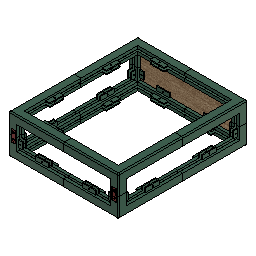
Frame_v46 (Autodesk Fusion 360 design; units mm, degrees)
Autodesk Fusion 360 part; units mm, degrees
(part 1 of 4)
sketch "Esquisse1" plane through (0, 0, 0) normal (0, 0, 1) x (1, 0, 0) in component "Wood_Bottom"
  line L0 (-125, 150) -> (125, 150)
  line L1 (125, 150) -> (125, -150)
  line L2 (125, -150) -> (-125, -150)
  line L3 (-125, -150) -> (-125, 150)
  line L4 (0, 150) -> (0, -150) construction
  line L5 (-125, 0) -> (125, 0) construction
  dimension "d4" = 250
  dimension "d5" = 300
  constraint horizontal L0
  constraint vertical L1
  constraint horizontal L2
  constraint vertical L3
  constraint midpoint L0 L4.start
  constraint midpoint L2 L4.end
  constraint midpoint L3 L5.start
  constraint midpoint L1 L5.end
  constraint midpoint L4 origin
  measures "d4" distance of L0.start L0.end
  measures "d5" distance of L0.start L2.end
extrude "Extrusion1" add sketch "Esquisse1" along normal blind 5 makes body 1 in component "Wood_Bottom"
sketch "Esquisse1 (2)" plane through (0, 0, 0) normal (1, 0, 0) x (0, 1, 0) in component "Right_Bottom_Holder"
  line L0 (-165, 59.7937) -> (165, 59.7937)
  line L1 (165, 59.7937) -> (165, 39.4937)
  line L2 (165, 39.4937) -> (-165, 39.4937)
  line L3 (-165, 39.4937) -> (-165, 59.7937)
  line L4 (0, 59.7937) -> (0, 39.4937) construction
  line L5 (-165, 49.6437) -> (165, 49.6437) construction
  point P0 (0, 49.6437)
  dimension "d11" = 330
  dimension "d12" = 20.3
  constraint horizontal L0
  constraint vertical L1
  constraint horizontal L2
  constraint vertical L3
  constraint midpoint L0 L4.start
  constraint midpoint L2 L4.end
  constraint midpoint L3 L5.start
  constraint midpoint L1 L5.end
  constraint midpoint L5 P0
  constraint vertical origin P0
  measures "d11" distance of L0.start L0.end
  measures "d12" distance of L0.start L2.end
extrude "Extrusion1'" add sketch "Esquisse1 (2)" along normal blind 20 separate body makes body 2 in component "Right_Bottom_Holder"
sketch "Esquisse2" plane through (0, 0, 0) normal (-1, 0, 0) x (0, -1, 0) in component "Right_Bottom_Holder"
  line L0 (-165, 39.4937) -> (165, 39.4937)
  line L1 (165, 39.4937) -> (165, 59.7937)
  line L2 (165, 59.7937) -> (-165, 59.7937)
  line L3 (-165, 59.7937) -> (-165, 39.4937)
  line L4 (-150.3, 52.4437) -> (150.3, 52.4437)
  line L5 (150.3, 52.4437) -> (150.3, 46.8437)
  line L6 (150.3, 46.8437) -> (-150.3, 46.8437)
  line L7 (-150.3, 46.8437) -> (-150.3, 52.4437)
  line L8 (-165, 49.6437) -> (165, 49.6437) construction
  line L9 (0, 59.7937) -> (0, 39.4937) construction
  line L10 (-165, 59.7937) -> (-145, 59.7937)
  line L11 (-145, 59.7937) -> (-145, 39.4937)
  line L12 (-145, 39.4937) -> (-165, 39.4937)
  line L13 (-165, 39.4937) -> (-165, 59.7937)
  line L14 (165, 59.7937) -> (145, 59.7937)
  line L15 (145, 59.7937) -> (145, 39.4937)
  line L16 (145, 39.4937) -> (165, 39.4937)
  line L17 (165, 39.4937) -> (165, 59.7937)
  line L18 (90, 52.4437) -> (55, 52.4437)
  line L19 (55, 52.4437) -> (55, 54.9437)
  line L20 (55, 54.9437) -> (90, 54.9437)
  line L21 (90, 54.9437) -> (90, 52.4437)
  line L22 (90, 54.9437) -> (145, 54.9437) construction
  line L23 (55, 54.9437) -> (0, 54.9437) construction
  line L24 (90, 46.8437) -> (55, 46.8437)
  line L25 (90, 44.3437) -> (90, 46.8437)
  line L26 (55, 46.8437) -> (55, 44.3437)
  line L27 (55, 44.3437) -> (90, 44.3437)
  line L28 (-55, 46.8437) -> (-55, 44.3437)
  line L29 (-90, 54.9437) -> (-90, 52.4437)
  line L30 (-55, 52.4437) -> (-55, 54.9437)
  line L31 (-55, 54.9437) -> (-90, 54.9437)
  line L32 (-90, 44.3437) -> (-90, 46.8437)
  line L33 (-90, 46.8437) -> (-55, 46.8437)
  line L34 (-55, 44.3437) -> (-90, 44.3437)
  line L35 (-90, 52.4437) -> (-55, 52.4437)
  point P0 (150.3, 49.6437)
  point P1 (0, 52.4437)
  point P2 (0, 53.6937)
  dimension "d16" = 5.6
  dimension "d17" = 300.6
  dimension "d109" = 20
  dimension "d110" = 20.3
  dimension "d111" = 20
  dimension "d112" = 20.3
  dimension "d230" = 2.5
  dimension "d231" = 35
  constraint horizontal L4
  constraint vertical L5
  constraint horizontal L6
  constraint vertical L7
  constraint midpoint L3 L8.start
  constraint midpoint L1 L8.end
  constraint midpoint L5 P0
  constraint coincident L8 P0
  constraint midpoint L4 P1
  constraint midpoint L2 L9.start
  constraint midpoint L0 L9.end
  constraint coincident P1 L9
  constraint coincident L9 P2
  constraint horizontal L10
  constraint vertical L11
  constraint horizontal L12
  constraint vertical L13
  constraint coincident L2.end L3.start
  constraint horizontal L14
  constraint vertical L15
  constraint horizontal L16
  constraint vertical L17
  constraint coincident L1.end L2.start
  constraint horizontal L18
  constraint vertical L19
  constraint horizontal L20
  constraint vertical L21
  constraint coincident L4 L18.start
  constraint coincident L15 L22.end
  constraint perpendicular L15 L22
  constraint coincident L9 L23.end
  constraint perpendicular L9 L23
  constraint equal L22 L23
  constraint symmetric L8 L18.start L24.start
  constraint symmetric L8 L18.end L24.end
  constraint symmetric L8 L19.end L26.end
  constraint symmetric L8 L20.end L25.start
  constraint symmetric L9 L18.start L29.end
  constraint symmetric L9 L18.end L30.start
  constraint symmetric L9 L19.end L30.end
  constraint symmetric L9 L20.end L29.start
  constraint symmetric L9 L24.start L32.end
  constraint symmetric L9 L24.end L28.start
  constraint symmetric L9 L25.start L32.start
  constraint symmetric L9 L26.end L28.end
  measures "d16" distance of L4 L6
  measures "d17" distance of L4.start L4.end
  measures "d109" distance of L2.end L10.end
  measures "d110" distance of L10.end L11.end
  measures "d111" distance of L1.end L14.end
  measures "d112" distance of L14.end L15.end
  measures "d230" distance of L18.start L20.end
  measures "d231" distance of L19.end L20.end
extrude "Extrusion2" cut sketch "Esquisse2" against normal blind 5 contours L4 L6 L11 L15 L18 L24 L33 L35 | L4 L6 L7 L11 | L4 L5 L6 L15 bodies 2 in component "Right_Bottom_Holder"
extrude "Extrusion3" add sketch "Esquisse2" along normal blind 10 contours L6 L28 L32 L33 L34 | L6 L24 L25 L26 L27 | L4 L29 L30 L31 L35 | L4 L18 L19 L20 L21 bodies 2 in component "Right_Bottom_Holder"
extrude "Extrusion19" add sketch "Esquisse2" along normal blind 120.3 contours L0 L2 L3 L4 L6 L7 L10 L11 L12 L13 | L0 L1 L2 L4 L5 L6 L14 L15 L16 L17 bodies 2 in component "Right_Bottom_Holder"
sketch "Esquisse14" plane through (-120.3, 0, 0) normal (-1, 0, 0) x (0, -1, 0) in component "Right_Bottom_Holder"
  line L0 (-145, 46.8437) -> (-150.3, 46.8437)
  line L1 (-150.3, 46.8437) -> (-150.3, 52.4437)
  line L2 (-150.3, 52.4437) -> (-145, 52.4437)
  line L3 (-145, 52.4437) -> (-145, 59.7937)
  line L4 (-145, 59.7937) -> (-165, 59.7937)
  line L5 (-165, 59.7937) -> (-165, 39.4937)
  line L6 (-165, 39.4937) -> (-145, 39.4937)
  line L7 (-145, 39.4937) -> (-145, 46.8437)
  line L8 (-155, 59.7937) -> (-155, 39.4937) construction
  line L9 (-165, 49.6437) -> (-155, 49.6437) construction
  line L10 (-165, 49.6437) -> (-155, 39.4937) construction
  line L11 (-165, 39.4937) -> (-155, 49.6437) construction
  circle A0 centre (-160, 44.5687) radius 2.65
  line L12 (-157.8, 59.7937) -> (-152.2, 59.7937)
  line L13 (-152.2, 59.7937) -> (-152.2, 54.4937)
  line L14 (-152.2, 54.4937) -> (-157.8, 54.4937)
  line L15 (-157.8, 54.4937) -> (-157.8, 59.7937)
  point P0 (-155, 54.4937)
  dimension "d117" = 5.3
  dimension "d118" = 5.6
  dimension "d119" = 5.3
  constraint midpoint L4 L8.start
  constraint midpoint L6 L8.end
  constraint midpoint L5 L9.start
  constraint midpoint L8 L9.end
  constraint coincident L5.end L6.start
  constraint midpoint L10 A0.centre
  constraint horizontal L12
  constraint vertical L13
  constraint horizontal L14
  constraint vertical L15
  constraint coincident L4 L12.start
  constraint midpoint L14 P0
  constraint coincident L8 P0
  measures "d117" diameter of A0
  measures "d118" distance of L13.end L14.end
  measures "d119" distance of L12.end L13.end
extrude "Extrusion20" cut sketch "Esquisse14" against normal blind 10.3 contours A0 bodies 2 in component "Right_Bottom_Holder"
extrude "Extrusion21" cut sketch "Esquisse14" against normal up to surface (125.6 mm away) contours L4 L12 L13 L14 L15 bodies 2 in component "Right_Bottom_Holder"
sketch "Esquisse15" plane through (0, 145, 0) normal (0, -1, 0) x (1, 0, 0) in component "Right_Bottom_Holder"
  line L0 (0, 52.4437) -> (0, 59.7937)
  line L1 (0, 59.7937) -> (-120.3, 59.7937)
  line L2 (-120.3, 59.7937) -> (-120.3, 52.4437)
  line L3 (-120.3, 52.4437) -> (0, 52.4437)
  line L4 (0, 46.8437) -> (-120.3, 46.8437)
  line L5 (-120.3, 46.8437) -> (-120.3, 39.4937)
  line L6 (-120.3, 39.4937) -> (0, 39.4937)
  line L7 (-60.15, 59.7937) -> (-60.15, 52.4437) construction
  line L8 (-60.15, 52.4437) -> (-60.15, 46.8437) construction
  line L9 (-60.15, 49.6437) -> (-55, 49.6437) construction
  line L10 (-77.65, 52.4437) -> (-42.65, 52.4437)
  line L11 (-42.65, 52.4437) -> (-42.65, 54.9437)
  line L12 (-42.65, 54.9437) -> (-77.65, 54.9437)
  line L13 (-77.65, 54.9437) -> (-77.65, 52.4437)
  line L14 (-42.65, 44.3437) -> (-77.65, 44.3437)
  line L15 (-77.65, 44.3437) -> (-77.65, 46.8437)
  line L16 (-77.65, 46.8437) -> (-42.65, 46.8437)
  line L17 (-42.65, 46.8437) -> (-42.65, 44.3437)
  line L18 (0, 39.4937) -> (0, 46.8437)
  point P0 (-60.15, 54.9437)
  dimension "d124" = 2.5
  dimension "d125" = 35
  constraint midpoint L1 L7.start
  constraint midpoint L3 L7.end
  constraint midpoint L4 L8.end
  constraint midpoint L8 L9.start
  constraint perpendicular L8 L9
  constraint horizontal L10
  constraint vertical L11
  constraint horizontal L12
  constraint vertical L13
  constraint coincident L3 L10.start
  constraint midpoint L12 P0
  constraint coincident L7 P0
  constraint symmetric L9 L10.start L15.end
  constraint symmetric L9 L10.end L16.end
  constraint symmetric L9 L11.end L14.start
  constraint symmetric L9 L12.end L14.end
  measures "d124" distance of L10.end L11.end
  measures "d125" distance of L11.end L12.end
extrude "Extrusion22" add sketch "Esquisse15" along normal blind 10 contours L3 L10 L11 L12 L13 | L4 L14 L15 L16 L17 bodies 2 in component "Right_Bottom_Holder"
sketch "Esquisse17" plane through (-120.3, 0, 0) normal (-1, 0, 0) x (0, -1, 0) in component "Right_Bottom_Holder"
  line L0 (165, 39.4937) -> (165, 59.7937)
  line L1 (165, 59.7937) -> (145, 59.7937)
  line L2 (145, 59.7937) -> (145, 52.4437)
  line L3 (145, 52.4437) -> (150.3, 52.4437)
  line L4 (150.3, 52.4437) -> (150.3, 46.8437)
  line L5 (150.3, 46.8437) -> (145, 46.8437)
  line L6 (145, 46.8437) -> (145, 39.4937)
  line L7 (145, 39.4937) -> (165, 39.4937)
  line L8 (155, 59.7937) -> (155, 39.4937) construction
  line L9 (165, 49.6437) -> (145, 49.6437) construction
  line L10 (155, 49.6437) -> (165, 39.4937) construction
  line L11 (155, 39.4937) -> (165, 49.6437) construction
  circle A0 centre (160, 44.5687) radius 2.65
  line L12 (152.2, 59.7937) -> (157.8, 59.7937)
  line L13 (157.8, 59.7937) -> (157.8, 54.4937)
  line L14 (157.8, 54.4937) -> (152.2, 54.4937)
  line L15 (152.2, 54.4937) -> (152.2, 59.7937)
  point P0 (155, 54.4937)
  dimension "d134" = 5.3
  dimension "d135" = 5.3
  dimension "d136" = 5.6
  constraint midpoint L1 L8.start
  constraint midpoint L7 L8.end
  constraint midpoint L0 L9.start
  constraint perpendicular L2 L9
  constraint midpoint L8 L10.start
  constraint coincident L0.start L7.end
  constraint midpoint L10 A0.centre
  constraint horizontal L12
  constraint vertical L13
  constraint horizontal L14
  constraint vertical L15
  constraint coincident L1 L12.start
  constraint midpoint L14 P0
  constraint coincident L8 P0
  measures "d134" diameter of A0
  measures "d135" distance of L12.end L13.end
  measures "d136" distance of L13.end L14.end
extrude "Extrusion25" cut sketch "Esquisse17" against normal blind 10.3 contours A0 bodies 2 in component "Right_Bottom_Holder"
extrude "Extrusion26" cut sketch "Esquisse17" against normal up to surface (125.6 mm away) contours L1 L12 L13 L14 L15 bodies 2 in component "Right_Bottom_Holder"
sketch "Esquisse18" plane through (0, -145, 0) normal (0, 1, 0) x (-1, 0, 0) in component "Right_Bottom_Holder"
  line L0 (0, 59.7937) -> (0, 52.4437)
  line L1 (0, 52.4437) -> (120.3, 52.4437)
  line L2 (120.3, 52.4437) -> (120.3, 59.7937)
  line L3 (120.3, 59.7937) -> (0, 59.7937)
  line L4 (0, 39.4937) -> (120.3, 39.4937) construction
  line L5 (120.3, 39.4937) -> (120.3, 46.8437) construction
  line L6 (120.3, 46.8437) -> (0, 46.8437) construction
  line L7 (60.15, 59.7937) -> (60.15, 52.4437) construction
  line L8 (60.15, 52.4437) -> (60.15, 46.8437) construction
  line L9 (60.15, 49.6437) -> (66.8882, 49.6437) construction
  line L10 (42.65, 52.4437) -> (77.65, 52.4437)
  line L11 (77.65, 52.4437) -> (77.65, 54.9437)
  line L12 (77.65, 54.9437) -> (42.65, 54.9437)
  line L13 (42.65, 54.9437) -> (42.65, 52.4437)
  line L14 (77.65, 44.3437) -> (42.65, 44.3437)
  line L15 (77.65, 46.8437) -> (77.65, 44.3437)
  line L16 (42.65, 44.3437) -> (42.65, 46.8437)
  line L17 (42.65, 46.8437) -> (77.65, 46.8437)
  line L18 (0, 46.8437) -> (0, 39.4937)
  point P0 (60.15, 54.9437)
  dimension "d141" = 2.5
  dimension "d142" = 35
  constraint midpoint L3 L7.start
  constraint midpoint L1 L7.end
  constraint midpoint L6 L8.end
  constraint midpoint L8 L9.start
  constraint perpendicular L8 L9
  constraint horizontal L10
  constraint vertical L11
  constraint horizontal L12
  constraint vertical L13
  constraint coincident L1 L10.start
  constraint midpoint L12 P0
  constraint coincident L7 P0
  constraint symmetric L9 L10.start L16.end
  constraint symmetric L9 L10.end L15.start
  constraint symmetric L9 L11.end L14.start
  constraint symmetric L9 L12.end L14.end
  measures "d141" distance of L10.end L11.end
  measures "d142" distance of L11.end L12.end
extrude "Extrusion27" add sketch "Esquisse18" along normal blind 10 contours L1 L10 L11 L12 L13 | L14 L15 L16 L17 bodies 2 in component "Right_Bottom_Holder"
sketch "Esquisse16" plane through (0, 0, 59.7937) normal (0, 0, 1) x (-1, 0, 0) in component "Right_Bottom_Holder"
  line L0 (-5.3, -152.2) -> (120.3, -152.2)
  line L1 (120.3, -152.2) -> (120.3, -145)
  line L2 (120.3, -145) -> (0, -145)
  line L3 (0, -145) -> (0, 145)
  line L4 (0, 145) -> (120.3, 145)
  line L5 (120.3, 157.8) -> (120.3, 165)
  line L6 (120.3, 165) -> (-20, 165)
  line L7 (-20, 165) -> (-20, -165)
  line L8 (-20, -165) -> (120.3, -165)
  line L9 (120.3, -165) -> (120.3, -157.8)
  line L10 (120.3, -157.8) -> (-5.3, -157.8)
  line L11 (-5.3, -157.8) -> (-5.3, -152.2)
  line L12 (0.0045, -165) -> (120.3, -165) construction
  line L13 (60.1522, -165) -> (60.15, -145) construction
  line L14 (60.1511, -155) -> (47.2609, -155.0014) construction
  line L15 (77.6517, -157.8) -> (42.6517, -157.8)
  line L16 (42.6517, -157.8) -> (42.6517, -160.3)
  line L17 (42.6517, -160.3) -> (77.6517, -160.3)
  line L18 (77.6517, -160.3) -> (77.6517, -157.8)
  line L19 (77.6505, -149.6961) -> (77.6511, -152.1961)
  line L20 (42.6505, -149.7039) -> (77.6505, -149.6961)
  line L21 (77.6511, -152.1961) -> (42.6511, -152.2039)
  line L22 (42.6511, -152.2039) -> (42.6505, -149.7039)
  line L23 (0, -145) -> (-20, -145)
  line L24 (-20, -145) -> (-20, -165)
  line L25 (-20, -165) -> (0, -165)
  line L26 (0, -165) -> (0, -145)
  line L27 (-20, 0) -> (0, 0) construction
  line L28 (-12.8, -150.3) -> (-7.2, -150.3)
  line L29 (-7.2, -150.3) -> (-7.2, 150.3)
  line L30 (-7.2, 150.3) -> (-12.8, 150.3)
  line L31 (-12.8, 150.3) -> (-12.8, -150.3)
  line L32 (-10, -165) -> (-10, -145) construction
  line L33 (0, 145) -> (-20, 145)
  line L34 (-20, 145) -> (-20, 165)
  line L35 (-20, 165) -> (0, 165)
  line L36 (0, 165) -> (0, 145)
  line L37 (-12.8, 70) -> (-12.8, -70)
  line L38 (-10, 0) -> (-10, 10) construction
  line L39 (-7.2, 70) -> (-7.2, -70)
  line L40 (0, 165) -> (120.3, 165) construction
  line L41 (60.15, 165) -> (60.15, 145) construction
  line L42 (-5.3, 157.8) -> (120.3, 157.8)
  line L43 (120.3, 152.2) -> (-5.3, 152.2)
  line L44 (-5.3, 152.2) -> (-5.3, 157.8)
  line L45 (-5.3, 157.8) -> (-5.3, 152.2)
  line L46 (-5.3, 152.2) -> (120.3, 152.2)
  line L47 (120.3, 152.2) -> (120.3, 157.8)
  line L48 (120.3, 157.8) -> (-5.3, 157.8)
  line L49 (42.65, 157.8) -> (77.65, 157.8)
  line L50 (77.65, 157.8) -> (77.65, 160.3)
  line L51 (77.65, 160.3) -> (42.65, 160.3)
  line L52 (42.65, 160.3) -> (42.65, 157.8)
  line L53 (60.15, 155) -> (66, 155) construction
  line L54 (42.65, 152.2) -> (77.65, 152.2)
  line L55 (42.65, 149.7) -> (42.65, 152.2)
  line L56 (77.65, 149.7) -> (42.65, 149.7)
  line L57 (77.65, 152.2) -> (77.65, 149.7)
  line L58 (-12.8, -90) -> (-15.3, -90)
  line L59 (-15.3, -90) -> (-15.3, -55)
  line L60 (-15.3, -55) -> (-12.8, -55)
  line L61 (-12.8, -55) -> (-12.8, -90)
  line L62 (-15.3, -90) -> (-15.3, -145) construction
  line L63 (-15.3, -55) -> (-15.3, 0) construction
  line L64 (-4.7, -90) -> (-4.7, -55)
  line L65 (-4.7, -55) -> (-7.2, -55)
  line L66 (-7.2, -90) -> (-4.7, -90)
  line L67 (-7.2, -55) -> (-7.2, -90)
  line L68 (-7.2, 55) -> (-7.2, 90)
  line L69 (-12.8, 55) -> (-12.8, 90)
  line L70 (-15.3, 55) -> (-12.8, 55)
  line L71 (-15.3, 90) -> (-15.3, 55)
  line L72 (-12.8, 90) -> (-15.3, 90)
  line L73 (-7.2, 90) -> (-4.7, 90)
  line L74 (-4.7, 90) -> (-4.7, 55)
  line L75 (-4.7, 55) -> (-7.2, 55)
  point P0 (60.1517, -160.3)
  point P1 (-10, -150.3)
  point P2 (-12.8, 0)
  point P3 (-15.3, 0)
  point P4 (60.15, 160.3)
  dimension "d128" = 2.5
  dimension "d129" = 35
  dimension "d145" = 5.6
  dimension "d146" = 300.6
  dimension "d149" = 2.5
  dimension "d150" = 35
  dimension "d232" = 2.5
  dimension "d233" = 35
  constraint coincident L8 L12.start
  constraint coincident L8.end L9.start
  constraint midpoint L12 L13.start
  constraint midpoint L2 L13.end
  constraint midpoint L13 L14.start
  constraint perpendicular L13 L14
  constraint horizontal L15
  constraint vertical L16
  constraint horizontal L17
  constraint vertical L18
  constraint coincident L10 L15.start
  constraint midpoint L17 P0
  constraint coincident L13 P0
  constraint symmetric L14 L15.start L19.end
  constraint symmetric L14 L15.end L21.end
  constraint symmetric L14 L16.end L20.start
  constraint symmetric L14 L17.end L19.start
  constraint horizontal L23
  constraint vertical L24
  constraint horizontal L25
  constraint vertical L26
  constraint coincident L7.end L8.start
  constraint coincident L2.end L3.start
  constraint midpoint L7 L27.start
  constraint coincident L27.end origin
  constraint horizontal L28
  constraint vertical L29
  constraint horizontal L30
  constraint vertical L31
  constraint midpoint L28 P1
  constraint midpoint L25 L32.start
  constraint midpoint L23 L32.end
  constraint coincident P1 L32
  constraint midpoint L31 P2
  constraint coincident L27 P2
  constraint horizontal L33
  constraint vertical L34
  constraint horizontal L35
  constraint vertical L36
  constraint coincident L6.end L7.start
  constraint coincident L3.end L4.start
  constraint vertical L37
  constraint coincident L31 L37.end
  constraint coincident L27 P3
  constraint midpoint L27 L38.start
  constraint perpendicular L27 L38
  constraint symmetric L37.end L38 L39.end
  constraint symmetric L37.start L38 L39.start
  constraint coincident L5.end L6.start
  constraint midpoint L40 L41.start
  constraint midpoint L4 L41.end
  constraint horizontal L49
  constraint vertical L50
  constraint horizontal L51
  constraint vertical L52
  constraint coincident L42 L49.start
  constraint midpoint L51 P4
  constraint coincident L41 P4
  constraint midpoint L41 L53.start
  constraint perpendicular L41 L53
  constraint symmetric L49.start L53 L54.start
  constraint symmetric L49.end L53 L54.end
  constraint symmetric L50.end L53 L56.start
  constraint symmetric L51.end L53 L55.start
  constraint horizontal L58
  constraint vertical L59
  constraint horizontal L60
  constraint vertical L61
  constraint coincident L31 L58.start
  constraint coincident L23 L62.end
  constraint perpendicular L23 L62
  constraint coincident P3 L63.end
  constraint perpendicular L27 L63
  constraint equal L62 L63
  constraint symmetric L38 L58.start L66.start
  constraint symmetric L38 L58.end L64.start
  constraint symmetric L38 L59.end L64.end
  constraint symmetric L38 L60.end L65.end
  constraint symmetric L27 L58.start L69.end
  constraint symmetric L27 L58.end L71.start
  constraint symmetric L27 L59.end L70.start
  constraint symmetric L27 L60.end L69.start
  constraint symmetric L27 L64.start L73.end
  constraint symmetric L27 L64.end L74.end
  constraint symmetric L27 L65.end L68.start
  constraint symmetric L27 L66.start L68.end
  measures "d128" distance of L15.end L16.end
  measures "d129" distance of L16.end L17.end
  measures "d145" distance of L28.start L28.end
  measures "d146" distance of L28.start L30.end
  measures "d149" distance of L49.start L51.end
  measures "d150" distance of L50.end L51.end
  measures "d232" distance of L58.start L58.end
  measures "d233" distance of L58.end L59.end
extrude "Extrusion23" add sketch "Esquisse16" along normal blind 10 contours L0 L19 L20 L21 L22 | L0 L21 L22 | L10 L15 L16 L17 L18 | L29 L39 L64 L65 L66 L67 | L29 L39 L68 L73 L74 L75 | L43 L46 L54 L55 L56 L57 | L31 L37 L58 L59 L60 L61 | L31 L37 L69 L70 L71 L72 | L42 L48 L49 L50 L51 L52 bodies 2 in component "Right_Bottom_Holder"
extrude "Extrusion28" cut sketch "Esquisse16" against normal blind 5.3 contours L23 L28 L29 L31 | L23 L29 L31 L33 L37 L39 L61 L67 L68 L69 | L29 L30 L31 L33 bodies 2 in component "Right_Bottom_Holder"
extrude "Extrusion29" add sketch "Esquisse16" along normal blind 30 contours L0 L7 L8 L10 L11 L23 L24 L25 L26 L28 L29 L31 | L6 L7 L29 L30 L31 L33 L34 L35 L36 L42 L43 L44 L45 L46 L48 bodies 2 in component "Right_Bottom_Holder"
sketch "Esquisse20" plane through (0, 0, 89.7937) normal (0, 0, 1) x (-1, 0, 0) in component "Right_Bottom_Holder"
  line L0 (0, 165) -> (-20, 165)
  line L1 (-20, 165) -> (-20, 145)
  line L2 (-20, 145) -> (-12.8, 145)
  line L3 (-12.8, 145) -> (-12.8, 150.3)
  line L4 (-12.8, 150.3) -> (-7.2, 150.3)
  line L5 (-7.2, 150.3) -> (-7.2, 145)
  line L6 (-7.2, 145) -> (0, 145)
  line L7 (0, 145) -> (0, 152.2)
  line L8 (0, 152.2) -> (-5.3, 152.2)
  line L9 (-5.3, 152.2) -> (-5.3, 157.8)
  line L10 (-5.3, 157.8) -> (0, 157.8)
  line L11 (0, 157.8) -> (0, 165)
  line L12 (-20, 155) -> (0, 155) construction
  line L13 (-10, 165) -> (-10, 145) construction
  circle A0 centre (-15, 155) radius 2.5
  line L14 (-20, 145) -> (0, 145) construction
  line L15 (-20, 165) -> (-10, 165) construction
  line L16 (-15, 165) -> (-15, 145) construction
  line L17 (-12.8, -150.3) -> (-12.8, -145)
  line L18 (-12.8, -145) -> (-20, -145)
  line L19 (-20, -145) -> (-20, -165)
  line L20 (-20, -165) -> (0, -165)
  line L21 (0, -165) -> (0, -157.8)
  line L22 (0, -157.8) -> (-5.3, -157.8)
  line L23 (-5.3, -157.8) -> (-5.3, -152.2)
  line L24 (-5.3, -152.2) -> (0, -152.2)
  line L25 (0, -152.2) -> (0, -145)
  line L26 (0, -145) -> (-7.2, -145)
  line L27 (-7.2, -145) -> (-7.2, -150.3)
  line L28 (-7.2, -150.3) -> (-12.8, -150.3)
  line L29 (-10, -165) -> (-10, -145) construction
  line L30 (-20, -155) -> (0, -155) construction
  line L31 (-10, -165) -> (-20, -165) construction
  line L32 (-15, -165) -> (-15, -145) construction
  circle A1 centre (-15, -155) radius 2.5
  dimension "d158" = 5
  dimension "d352" = 10
  dimension "d354" = 5
  constraint midpoint L1 L12.start
  constraint perpendicular L7 L12
  constraint midpoint L0 L13.start
  constraint perpendicular L2 L13
  constraint coincident L0.end L1.start
  constraint coincident L1.end L2.start
  constraint coincident L6.end L7.start
  constraint midpoint L15 L16.start
  constraint coincident L14 L16.end
  constraint coincident A0.centre L16
  constraint midpoint L20 L29.start
  constraint perpendicular L26 L29
  constraint midpoint L19 L30.start
  constraint perpendicular L23 L30
  constraint coincident L19.end L20.start
  constraint midpoint L31 L32.start
  constraint coincident L18 L32.end
  constraint perpendicular L18 L32
  constraint midpoint L32 A1.centre
  measures "d158" diameter of A0
  measures "d352" distance of A0.centre L15
  measures "d354" diameter of A1
extrude "Extrusion31" add sketch "Esquisse20" along normal blind 10 contours A0 | A1 bodies 2 in component "Right_Bottom_Holder"
split "Scinder1" by plane through (-120.3, 0, 47.1437) normal (0, 1, 0) bodies 2 makes body 3 at (13.3333, 103.3333, 39.4937) in component "Right_Bottom_Holder"
move_body "Déplacer1" bodies 2 to x (1, 0, 0) y (0, 1, 0) z (0, 0, 1) at (0, -80, 0) in component "Right_Bottom_Holder"
sketch "Esquisse21" plane through (0, -80, 0) normal (0, 1, 0) x (-1, 0, 0) in component "Right_Bottom_Holder"
  line L0 (-10, 39.7937) -> (-10, 54.4937) construction
  line L1 (-20, 49.7937) -> (-5, 49.7937) construction
  line L2 (-20, 49.7937) -> (-10, 39.7937) construction
  line L3 (-10, 49.7937) -> (-20, 39.7937) construction
  circle A0 centre (-15, 44.7937) radius 2.65
  line L4 (0, 39.4937) -> (0, 46.8437)
  line L5 (0, 46.8437) -> (-5, 46.8437)
  line L6 (-5, 46.8437) -> (-5, 52.4437)
  line L7 (-5, 52.4437) -> (0, 52.4437)
  line L8 (0, 52.4437) -> (0, 59.7937)
  line L9 (0, 59.7937) -> (-7.2, 59.7937)
  line L10 (-7.2, 59.7937) -> (-7.2, 54.4937)
  line L11 (-7.2, 54.4937) -> (-12.8, 54.4937)
  line L12 (-12.8, 54.4937) -> (-12.8, 59.7937)
  line L13 (-12.8, 59.7937) -> (-20, 59.7937)
  line L14 (-20, 59.7937) -> (-20, 39.4937)
  line L15 (-20, 39.4937) -> (0, 39.4937)
  dimension "d161" = 5.3
  constraint coincident L0 L3.start
  constraint coincident L1 L3.start
  constraint midpoint L3 A0.centre
  measures "d161" diameter of A0
extrude "Extrusion32" cut sketch "Esquisse21" against normal blind 10.3 contours A0 bodies 2 in component "Right_Bottom_Holder"
sketch "Esquisse22" plane through (0, 0, 0) normal (0, -1, 0) x (1, 0, 0) in component "Right_Bottom_Holder"
  line L0 (10, 39.7937) -> (10, 54.4937) construction
  line L1 (20, 49.7937) -> (5, 49.7937) construction
  line L2 (20, 39.7937) -> (10, 49.7937) construction
  line L3 (10, 39.7937) -> (20, 49.7937) construction
  circle A0 centre (15, 44.7937) radius 2.5
  line L4 (0, 46.8437) -> (0, 39.4937)
  line L5 (0, 39.4937) -> (20, 39.4937)
  line L6 (20, 39.4937) -> (20, 59.7937)
  line L7 (20, 59.7937) -> (12.8, 59.7937)
  line L8 (12.8, 59.7937) -> (12.8, 54.4937)
  line L9 (12.8, 54.4937) -> (7.2, 54.4937)
  line L10 (7.2, 54.4937) -> (7.2, 59.7937)
  line L11 (7.2, 59.7937) -> (0, 59.7937)
  line L12 (0, 59.7937) -> (0, 52.4437)
  line L13 (0, 52.4437) -> (5, 52.4437)
  line L14 (5, 52.4437) -> (5, 46.8437)
  line L15 (5, 46.8437) -> (0, 46.8437)
  dimension "d164" = 5
  constraint coincident L1 L2.end
  constraint coincident L0 L2.end
  constraint midpoint L3 A0.centre
  measures "d164" diameter of A0
extrude "Extrusion33" add sketch "Esquisse22" along normal blind 10 contours A0 bodies 3 in component "Right_Bottom_Holder"
move_body "Déplacer2" bodies 2 to x (1, 0, 0) y (0, 1, 0) z (0, 0, 1) at (0, 80, 0) in component "Right_Bottom_Holder"
sketch "Esquisse23" plane through (0, 145, 0) normal (0, -1, 0) x (1, 0, 0) in component "Right_Bottom_Holder"
  line L0 (0, 59.7937) -> (7.2, 59.7937)
  line L1 (7.2, 59.7937) -> (7.2, 89.7937)
  line L2 (7.2, 89.7937) -> (0, 89.7937)
  line L3 (0, 89.7937) -> (0, 59.7937)
  line L4 (12.8, 59.7937) -> (20, 59.7937)
  line L5 (20, 59.7937) -> (20, 89.7937)
  line L6 (20, 89.7937) -> (12.8, 89.7937)
  line L7 (12.8, 89.7937) -> (12.8, 59.7937)
  line L8 (0, 74.7937) -> (7.2, 74.7937) construction
  line L9 (7.2, 74.7937) -> (12.8, 74.7937) construction
  line L10 (10, 74.7937) -> (10, 86.5) construction
  line L11 (7.2, 66.0437) -> (4.7, 66.0437)
  line L12 (4.7, 66.0437) -> (4.7, 83.5437)
  line L13 (4.7, 83.5437) -> (7.2, 83.5437)
  line L14 (7.2, 83.5437) -> (7.2, 66.0437)
  line L15 (15.3, 66.0437) -> (15.3, 83.5437)
  line L16 (15.3, 83.5437) -> (12.8, 83.5437)
  line L17 (12.8, 83.5437) -> (12.8, 66.0437)
  line L18 (12.8, 66.0437) -> (15.3, 66.0437)
  point P0 (4.7, 74.7937)
  dimension "d171" = 2.5
  dimension "d172" = 17.5
  constraint midpoint L3 L8.start
  constraint midpoint L1 L8.end
  constraint midpoint L7 L9.end
  constraint midpoint L9 L10.start
  constraint perpendicular L9 L10
  constraint horizontal L11
  constraint vertical L12
  constraint horizontal L13
  constraint vertical L14
  constraint coincident L1 L11.start
  constraint midpoint L12 P0
  constraint coincident L8 P0
  constraint symmetric L10 L11.start L17.end
  constraint symmetric L10 L11.end L15.start
  constraint symmetric L10 L12.end L15.end
  constraint symmetric L10 L13.end L16.end
  measures "d171" distance of L12.end L13.end
  measures "d172" distance of L11.end L12.end
extrude "Extrusion35" add sketch "Esquisse23" along normal blind 10 contours L1 L11 L12 L13 L14 | L7 L15 L16 L17 L18 bodies 3 in component "Right_Bottom_Holder"
sketch "Esquisse24" plane through (0, -145, 0) normal (0, 1, 0) x (-1, 0, 0) in component "Right_Bottom_Holder"
  line L0 (-20, 59.7937) -> (-12.8, 59.7937)
  line L1 (-12.8, 59.7937) -> (-12.8, 89.7937)
  line L2 (-12.8, 89.7937) -> (-20, 89.7937)
  line L3 (-20, 89.7937) -> (-20, 59.7937)
  line L4 (-20, 74.7937) -> (-12.8, 74.7937) construction
  line L5 (-7.2, 59.7937) -> (0, 59.7937) construction
  line L6 (0, 59.7937) -> (0, 89.7937) construction
  line L7 (0, 89.7937) -> (-7.2, 89.7937) construction
  line L8 (-7.2, 89.7937) -> (-7.2, 59.7937) construction
  line L9 (-12.8, 74.7937) -> (-7.2, 74.7937) construction
  line L10 (-10, 74.7937) -> (-10, 87.5) construction
  line L11 (-12.8, 66.0437) -> (-15.3, 66.0437)
  line L12 (-15.3, 66.0437) -> (-15.3, 83.5437)
  line L13 (-15.3, 83.5437) -> (-12.8, 83.5437)
  line L14 (-12.8, 83.5437) -> (-12.8, 66.0437)
  line L15 (-4.7, 66.0437) -> (-4.7, 83.5437)
  line L16 (-4.7, 83.5437) -> (-7.2, 83.5437)
  line L17 (-7.2, 83.5437) -> (-7.2, 66.0437)
  line L18 (-7.2, 66.0437) -> (-4.7, 66.0437)
  point P0 (-15.3, 74.7937)
  dimension "d175" = 2.5
  dimension "d176" = 17.5
  constraint midpoint L3 L4.start
  constraint midpoint L1 L4.end
  constraint midpoint L8 L9.end
  constraint midpoint L9 L10.start
  constraint perpendicular L9 L10
  constraint horizontal L11
  constraint vertical L12
  constraint horizontal L13
  constraint vertical L14
  constraint coincident L1 L11.start
  constraint midpoint L12 P0
  constraint coincident L4 P0
  constraint symmetric L10 L11.start L17.end
  constraint symmetric L10 L11.end L15.start
  constraint symmetric L10 L12.end L15.end
  constraint symmetric L10 L13.end L16.end
  measures "d175" distance of L12.end L13.end
  measures "d176" distance of L11.end L12.end
extrude "Extrusion36" add sketch "Esquisse24" along normal blind 10 contours L1 L11 L12 L13 L14 | L15 L16 L17 L18 bodies 2 in component "Right_Bottom_Holder"
sketch "Esquisse1 (3)" plane through (0, 0, 0) normal (1, 0, 0) x (0, 1, 0) in component "Left_Bottom_Holder"
  line L0 (-165, 59.7937) -> (165, 59.7937)
  line L1 (165, 59.7937) -> (165, 39.4937)
  line L2 (165, 39.4937) -> (-165, 39.4937)
  line L3 (-165, 39.4937) -> (-165, 59.7937)
  line L4 (0, 59.7937) -> (0, 39.4937) construction
  line L5 (-165, 49.6437) -> (165, 49.6437) construction
  point P0 (0, 49.6437)
  dimension "d11_1" = 330
  dimension "d12_1" = 20.3
  constraint horizontal L0
  constraint vertical L1
  constraint horizontal L2
  constraint vertical L3
  constraint midpoint L0 L4.start
  constraint midpoint L2 L4.end
  constraint midpoint L3 L5.start
  constraint midpoint L1 L5.end
  constraint midpoint L5 P0
  constraint vertical origin P0
  measures "d11_1" distance of L0.start L0.end
  measures "d12_1" distance of L0.start L2.end
extrude "Extrusion1''" add sketch "Esquisse1 (3)" along normal blind 20 separate body makes body 4 in component "Left_Bottom_Holder"
sketch "Esquisse2 (2)" plane through (0, 0, 0) normal (-1, 0, 0) x (0, -1, 0) in component "Left_Bottom_Holder"
  line L0 (-165, 39.4937) -> (165, 39.4937)
  line L1 (165, 39.4937) -> (165, 59.7937)
  line L2 (165, 59.7937) -> (-165, 59.7937)
  line L3 (-165, 59.7937) -> (-165, 39.4937)
  line L4 (-150.3, 52.4437) -> (150.3, 52.4437)
  line L5 (150.3, 52.4437) -> (150.3, 46.8437)
  line L6 (150.3, 46.8437) -> (-150.3, 46.8437)
  line L7 (-150.3, 46.8437) -> (-150.3, 52.4437)
  line L8 (-165, 49.6437) -> (165, 49.6437) construction
  line L9 (0, 59.7937) -> (0, 39.4937) construction
  line L10 (-165, 59.7937) -> (-145, 59.7937)
  line L11 (-145, 59.7937) -> (-145, 39.4937)
  line L12 (-145, 39.4937) -> (-165, 39.4937)
  line L13 (-165, 39.4937) -> (-165, 59.7937)
  line L14 (165, 59.7937) -> (145, 59.7937)
  line L15 (145, 59.7937) -> (145, 39.4937)
  line L16 (145, 39.4937) -> (165, 39.4937)
  line L17 (165, 39.4937) -> (165, 59.7937)
  line L18 (-90, 52.4437) -> (-55, 52.4437)
  line L19 (-55, 52.4437) -> (-55, 54.9437)
  line L20 (-55, 54.9437) -> (-90, 54.9437)
  line L21 (-90, 54.9437) -> (-90, 52.4437)
  line L22 (-90, 54.9437) -> (-145, 54.9437) construction
  line L23 (-55, 54.9437) -> (0, 54.9437) construction
  line L24 (-90, 46.8437) -> (-55, 46.8437)
  line L25 (-90, 44.3437) -> (-90, 46.8437)
  line L26 (-55, 44.3437) -> (-90, 44.3437)
  line L27 (-55, 46.8437) -> (-55, 44.3437)
  line L28 (55, 44.3437) -> (90, 44.3437)
  line L29 (55, 54.9437) -> (90, 54.9437)
  line L30 (90, 44.3437) -> (90, 46.8437)
  line L31 (55, 52.4437) -> (55, 54.9437)
  line L32 (55, 46.8437) -> (55, 44.3437)
  line L33 (90, 46.8437) -> (55, 46.8437)
  line L34 (90, 52.4437) -> (55, 52.4437)
  line L35 (90, 54.9437) -> (90, 52.4437)
  point P0 (150.3, 49.6437)
  point P1 (0, 52.4437)
  point P2 (0, 53.6937)
  dimension "d16_1" = 5.6
  dimension "d17_1" = 300.6
  dimension "d109_1" = 20
  dimension "d110_1" = 20.3
  dimension "d111_1" = 20
  dimension "d112_1" = 20.3
  dimension "d234" = 2.5
  dimension "d235" = 35
  constraint horizontal L4
  constraint vertical L5
  constraint horizontal L6
  constraint vertical L7
  constraint midpoint L3 L8.start
  constraint midpoint L1 L8.end
  constraint midpoint L5 P0
  constraint coincident L8 P0
  constraint midpoint L4 P1
  constraint midpoint L2 L9.start
  constraint midpoint L0 L9.end
  constraint coincident P1 L9
  constraint coincident L9 P2
  constraint horizontal L10
  constraint vertical L11
  constraint horizontal L12
  constraint vertical L13
  constraint coincident L2.end L3.start
  constraint horizontal L14
  constraint vertical L15
  constraint horizontal L16
  constraint vertical L17
  constraint coincident L1.end L2.start
  constraint horizontal L18
  constraint vertical L19
  constraint horizontal L20
  constraint vertical L21
  constraint coincident L4 L18.start
  constraint coincident L11 L22.end
  constraint perpendicular L11 L22
  constraint coincident L9 L23.end
  constraint perpendicular L9 L23
  constraint equal L22 L23
  constraint symmetric L8 L18.start L24.start
  constraint symmetric L8 L18.end L24.end
  constraint symmetric L8 L19.end L26.start
  constraint symmetric L8 L20.end L25.start
  constraint symmetric L9 L18.start L34.start
  constraint symmetric L9 L18.end L31.start
  constraint symmetric L9 L19.end L29.start
  constraint symmetric L9 L20.end L29.end
  constraint symmetric L9 L24.start L30.end
  constraint symmetric L9 L24.end L32.start
  constraint symmetric L9 L25.start L28.end
  constraint symmetric L9 L26.start L28.start
  measures "d16_1" distance of L4 L6
  measures "d17_1" distance of L4.start L4.end
  measures "d109_1" distance of L2.end L10.end
  measures "d110_1" distance of L10.end L11.end
  measures "d111_1" distance of L1.end L14.end
  measures "d112_1" distance of L14.end L15.end
  measures "d234" distance of L18.start L20.end
  measures "d235" distance of L19.end L20.end
extrude "Extrusion2'" cut sketch "Esquisse2 (2)" against normal blind 5 contours L4 L6 L11 L15 L18 L24 L33 L34 | L4 L6 L7 L11 | L4 L5 L6 L15 bodies 4 in component "Left_Bottom_Holder"
extrude "Extrusion3'" add sketch "Esquisse2 (2)" along normal blind 10 contours L6 L24 L25 L26 L27 | L6 L28 L30 L32 L33 | L4 L18 L19 L20 L21 | L4 L29 L31 L34 L35 bodies 4 in component "Left_Bottom_Holder"
extrude "Extrusion19'" add sketch "Esquisse2 (2)" along normal blind 120.3 contours L0 L2 L3 L4 L6 L7 L10 L11 L12 L13 | L0 L1 L2 L4 L5 L6 L14 L15 L16 L17 bodies 4 in component "Left_Bottom_Holder"
sketch "Esquisse14 (2)" plane through (-120.3, 0, 0) normal (-1, 0, 0) x (0, -1, 0) in component "Left_Bottom_Holder"
  line L0 (-145, 46.8437) -> (-150.3, 46.8437)
  line L1 (-150.3, 46.8437) -> (-150.3, 52.4437)
  line L2 (-150.3, 52.4437) -> (-145, 52.4437)
  line L3 (-145, 52.4437) -> (-145, 59.7937)
  line L4 (-145, 59.7937) -> (-165, 59.7937)
  line L5 (-165, 59.7937) -> (-165, 39.4937)
  line L6 (-165, 39.4937) -> (-145, 39.4937)
  line L7 (-145, 39.4937) -> (-145, 46.8437)
  line L8 (-155, 59.7937) -> (-155, 39.4937) construction
  line L9 (-165, 49.6437) -> (-155, 49.6437) construction
  line L10 (-165, 49.6437) -> (-155, 39.4937) construction
  line L11 (-165, 39.4937) -> (-155, 49.6437) construction
  circle A0 centre (-160, 44.5687) radius 2.5
  line L12 (-157.8, 59.7937) -> (-152.2, 59.7937)
  line L13 (-152.2, 59.7937) -> (-152.2, 54.4937)
  line L14 (-152.2, 54.4937) -> (-157.8, 54.4937)
  line L15 (-157.8, 54.4937) -> (-157.8, 59.7937)
  point P0 (-155, 54.4937)
  dimension "d117_1" = 5
  dimension "d118_1" = 5.6
  dimension "d119_1" = 5.3
  constraint midpoint L4 L8.start
  constraint midpoint L6 L8.end
  constraint midpoint L5 L9.start
  constraint midpoint L8 L9.end
  constraint coincident L5.end L6.start
  constraint midpoint L10 A0.centre
  constraint horizontal L12
  constraint vertical L13
  constraint horizontal L14
  constraint vertical L15
  constraint coincident L4 L12.start
  constraint midpoint L14 P0
  constraint coincident L8 P0
  measures "d117_1" diameter of A0
  measures "d118_1" distance of L13.end L14.end
  measures "d119_1" distance of L12.end L13.end
extrude "Extrusion20'" add sketch "Esquisse14 (2)" along normal blind 10 contours A0 bodies 4 in component "Left_Bottom_Holder"
extrude "Extrusion21'" cut sketch "Esquisse14 (2)" against normal up to surface (125.6 mm away) contours L4 L12 L13 L14 L15 bodies 4 in component "Left_Bottom_Holder"
sketch "Esquisse15 (2)" plane through (0, 145, 0) normal (0, -1, 0) x (1, 0, 0) in component "Left_Bottom_Holder"
  line L0 (0, 52.4437) -> (0, 59.7937)
  line L1 (0, 59.7937) -> (-120.3, 59.7937)
  line L2 (-120.3, 59.7937) -> (-120.3, 52.4437)
  line L3 (-120.3, 52.4437) -> (0, 52.4437)
  line L4 (0, 46.8437) -> (-120.3, 46.8437)
  line L5 (-120.3, 46.8437) -> (-120.3, 39.4937)
  line L6 (-120.3, 39.4937) -> (0, 39.4937)
  line L7 (-60.15, 59.7937) -> (-60.15, 52.4437) construction
  line L8 (-60.15, 52.4437) -> (-60.15, 46.8437) construction
  line L9 (-60.15, 49.6437) -> (-55, 49.6437) construction
  line L10 (-77.65, 52.4437) -> (-42.65, 52.4437)
  line L11 (-42.65, 52.4437) -> (-42.65, 54.9437)
  line L12 (-42.65, 54.9437) -> (-77.65, 54.9437)
  line L13 (-77.65, 54.9437) -> (-77.65, 52.4437)
  line L14 (-42.65, 44.3437) -> (-77.65, 44.3437)
  line L15 (-77.65, 44.3437) -> (-77.65, 46.8437)
  line L16 (-77.65, 46.8437) -> (-42.65, 46.8437)
  line L17 (-42.65, 46.8437) -> (-42.65, 44.3437)
  line L18 (0, 39.4937) -> (0, 46.8437)
  point P0 (-60.15, 54.9437)
  dimension "d124_1" = 2.5
  dimension "d125_1" = 35
  constraint midpoint L1 L7.start
  constraint midpoint L3 L7.end
  constraint midpoint L4 L8.end
  constraint midpoint L8 L9.start
  constraint perpendicular L8 L9
  constraint horizontal L10
  constraint vertical L11
  constraint horizontal L12
  constraint vertical L13
  constraint coincident L3 L10.start
  constraint midpoint L12 P0
  constraint coincident L7 P0
  constraint symmetric L9 L10.start L15.end
  constraint symmetric L9 L10.end L16.end
  constraint symmetric L9 L11.end L14.start
  constraint symmetric L9 L12.end L14.end
  measures "d124_1" distance of L10.end L11.end
  measures "d125_1" distance of L11.end L12.end
extrude "Extrusion22'" add sketch "Esquisse15 (2)" along normal blind 10 contours L3 L10 L11 L12 L13 | L4 L14 L15 L16 L17 bodies 4 in component "Left_Bottom_Holder"
sketch "Esquisse17 (2)" plane through (-120.3, 0, 0) normal (-1, 0, 0) x (0, -1, 0) in component "Left_Bottom_Holder"
  line L0 (165, 39.4937) -> (165, 59.7937)
  line L1 (165, 59.7937) -> (145, 59.7937)
  line L2 (145, 59.7937) -> (145, 52.4437)
  line L3 (145, 52.4437) -> (150.3, 52.4437)
  line L4 (150.3, 52.4437) -> (150.3, 46.8437)
  line L5 (150.3, 46.8437) -> (145, 46.8437)
  line L6 (145, 46.8437) -> (145, 39.4937)
  line L7 (145, 39.4937) -> (165, 39.4937)
  line L8 (155, 59.7937) -> (155, 39.4937) construction
  line L9 (165, 49.6437) -> (145, 49.6437) construction
  line L10 (155, 49.6437) -> (165, 39.4937) construction
  line L11 (155, 39.4937) -> (165, 49.6437) construction
  circle A0 centre (160, 44.5687) radius 2.5
  line L12 (152.2, 59.7937) -> (157.8, 59.7937)
  line L13 (157.8, 59.7937) -> (157.8, 54.4937)
  line L14 (157.8, 54.4937) -> (152.2, 54.4937)
  line L15 (152.2, 54.4937) -> (152.2, 59.7937)
  point P0 (155, 54.4937)
  dimension "d134_1" = 5
  dimension "d135_1" = 5.3
  dimension "d136_1" = 5.6
  constraint midpoint L1 L8.start
  constraint midpoint L7 L8.end
  constraint midpoint L0 L9.start
  constraint perpendicular L2 L9
  constraint midpoint L8 L10.start
  constraint coincident L0.start L7.end
  constraint midpoint L10 A0.centre
  constraint horizontal L12
  constraint vertical L13
  constraint horizontal L14
  constraint vertical L15
  constraint coincident L1 L12.start
  constraint midpoint L14 P0
  constraint coincident L8 P0
  measures "d134_1" diameter of A0
  measures "d135_1" distance of L12.end L13.end
  measures "d136_1" distance of L13.end L14.end
extrude "Extrusion25'" add sketch "Esquisse17 (2)" along normal blind 10 contours A0 bodies 4 in component "Left_Bottom_Holder"
extrude "Extrusion26'" cut sketch "Esquisse17 (2)" against normal up to surface (125.6 mm away) contours L1 L12 L13 L14 L15 bodies 4 in component "Left_Bottom_Holder"
sketch "Esquisse18 (2)" plane through (0, -145, 0) normal (0, 1, 0) x (-1, 0, 0) in component "Left_Bottom_Holder"
  line L0 (0, 59.7937) -> (0, 52.4437)
  line L1 (0, 52.4437) -> (120.3, 52.4437)
  line L2 (120.3, 52.4437) -> (120.3, 59.7937)
  line L3 (120.3, 59.7937) -> (0, 59.7937)
  line L4 (0, 39.4937) -> (120.3, 39.4937) construction
  line L5 (120.3, 39.4937) -> (120.3, 46.8437) construction
  line L6 (120.3, 46.8437) -> (0, 46.8437) construction
  line L7 (60.15, 59.7937) -> (60.15, 52.4437) construction
  line L8 (60.15, 52.4437) -> (60.15, 46.8437) construction
  line L9 (60.15, 49.6437) -> (66.8882, 49.6437) construction
  line L10 (42.65, 52.4437) -> (77.65, 52.4437)
  line L11 (77.65, 52.4437) -> (77.65, 54.9437)
  line L12 (77.65, 54.9437) -> (42.65, 54.9437)
  line L13 (42.65, 54.9437) -> (42.65, 52.4437)
  line L14 (77.65, 44.3437) -> (42.65, 44.3437)
  line L15 (77.65, 46.8437) -> (77.65, 44.3437)
  line L16 (42.65, 44.3437) -> (42.65, 46.8437)
  line L17 (42.65, 46.8437) -> (77.65, 46.8437)
  line L18 (0, 46.8437) -> (0, 39.4937)
  point P0 (60.15, 54.9437)
  dimension "d141_1" = 2.5
  dimension "d142_1" = 35
  constraint midpoint L3 L7.start
  constraint midpoint L1 L7.end
  constraint midpoint L6 L8.end
  constraint midpoint L8 L9.start
  constraint perpendicular L8 L9
  constraint horizontal L10
  constraint vertical L11
  constraint horizontal L12
  constraint vertical L13
  constraint coincident L1 L10.start
  constraint midpoint L12 P0
  constraint coincident L7 P0
  constraint symmetric L9 L10.start L16.end
  constraint symmetric L9 L10.end L15.start
  constraint symmetric L9 L11.end L14.start
  constraint symmetric L9 L12.end L14.end
  measures "d141_1" distance of L10.end L11.end
  measures "d142_1" distance of L11.end L12.end
extrude "Extrusion27'" add sketch "Esquisse18 (2)" along normal blind 10 contours L1 L10 L11 L12 L13 | L14 L15 L16 L17 bodies 4 in component "Left_Bottom_Holder"